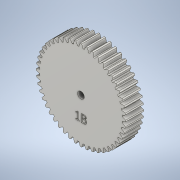
# Autodesk Inventor part: Spur Gear1
Saved by Autodesk Inventor 2021 (Build 250183000, 183)
## iProperties
CustomPartVersion: 0
Created: 2021-04-14
Part Number: Spur Gear1
Material: Steel
Document SubType Name: Modeling
Designer: Nabeel Azafer
Categories: <?xml version="1.0" encoding="UTF-16"?> <MemberInstance><Categories><FamilyTemplate><FamilyTemplateParameter ValueType="xs:double" Id="1" ObjectReferenceKey="da_z" ObjectType="kUserParameterObject"/><FamilyTemplateParameter ValueType="xs:double" Id="2" ObjectReferenceKey="da_b" ObjectType="kUserParameterObject"/><FamilyTemplateParameter ValueType="xs:double" Id="3" ObjectReferenceKey="da_beta" ObjectType="kUserParameterObject"/><FamilyTemplateParameter ValueType="xs:double" Id="4" ObjectReferenceKey="da_da" ObjectType="kUserParameterObject"/><FamilyTemplateParameter ValueType="xs:double" Id="5" ObjectReferenceKey="da_aw" ObjectType="kUserParameterObject"/><FamilyTemplateParameter ValueType="xs:string" Id="6" ObjectReferenceKey="EAIAABAAAACIAQAAAAAAAIAAAAAAAAAA" ObjectType="83910656" SubObjectId="SurfaceGeometry"/></FamilyTemplate><ParamToTemplateMap><ParamToTemplate CategoryParameter="//CategoryParameter[@InternalName='046C89C9-8512-4d59-83FE-43B91F4F132A']" TemplateParameter="1"/><ParamToTemplate CategoryParameter="//CategoryParameter[@InternalName='2552DF32-E462-4b46-AEBF-C6C7768E72AC']" TemplateParameter="2"/><ParamToTemplate CategoryParameter="//CategoryParameter[@InternalName='C9EE641D-15FC-4fae-A226-E94C4372FDD7']" TemplateParameter="3"/><ParamToTemplate><ParamToTemplate CategoryParameter="//CategoryParameter[@InternalName='00B6519A-459B-49c7-AD84-2E56D39A5744']" ConstantValue="0.000000"/></ParamToTemplate><ParamToTemplate><ParamToTemplate CategoryParameter="//CategoryParameter[@InternalName='04B31F0E-C7A6-4894-AA32-9629BEFACF47']" ConstantValue="0.800000"/></ParamToTemplate><ParamToTemplate><ParamToTemplate CategoryParameter="//CategoryParameter[@InternalName='43CBEC2E-7847-49e7-A936-2F7889FCB2D9']" ConstantValue="0.350000"/></ParamToTemplate><ParamToTemplate><ParamToTemplate CategoryParameter="//CategoryParameter[@InternalName='B1EFC894-105D-4ebd-86BF-FA20ED196853']" ConstantValue="0.500000"/></ParamToTemplate><ParamToTemplate><ParamToTemplate CategoryParameter="//CategoryParameter[@InternalName='51175063-3D10-4879-93E8-6246FE8B403D']" ConstantValue="2060000000.000000"/></ParamToTemplate><ParamToTemplate><ParamToTemplate CategoryParameter="//CategoryParameter[@InternalName='A3A52E27-4454-46a9-B0BD-C932399B70AF']" ConstantValue="0.300000"/></ParamToTemplate><ParamToTemplate><ParamToTemplate CategoryParameter="//CategoryParameter[@InternalName='91B76062-C214-41d9-B1B9-14D2AB99603D']" ConstantValue="0.080000"/></ParamToTemplate><ParamToTemplate><ParamToTemplate CategoryParameter="//CategoryParameter[@InternalName='374E806E-8B8A-4dda-A9AA-1039D6500AD2']" ConstantValue="12.500000"/></ParamToTemplate><ParamToTemplate><ParamToTemplate CategoryParameter="//CategoryParameter[@InternalName='2D373A89-B862-43d6-8D0B-0CBF12AB9F6C']" ConstantValue="0.349066"/></ParamToTemplate><ParamToTemplate CategoryParameter="//CategoryParameter[@InternalName='37777632-D6A2-4fac-9D53-DB8ACD95C989']" TemplateParameter="4"/><ParamToTemplate CategoryParameter="//CategoryParameter[@InternalName='FD1017F1-B727-4f7e-9707-0F86F1FF9423']" TemplateParameter="5"/><ParamToTemplate><ParamToTemplate CategoryParameter="//CategoryParameter[@InternalName='9E1B4470-B2D3-4ff1-B813-535BB4CDF51A']" ConstantValue="3520000.000000"/></ParamToTemplate><ParamToTemplate><ParamToTemplate CategoryParameter="//CategoryParameter[@InternalName='F8452263-BFF6-458c-9FB1-07C4B99E95CD']" ConstantValue="11400000.000000"/></ParamToTemplate><ParamToTemplate><ParamToTemplate CategoryParameter="//CategoryParameter[@InternalName='3E3BB259-FD49-497f-8171-6EBC954A3479']" ConstantValue="2.000000"/></ParamToTemplate><ParamToTemplate CategoryParameter="//CategoryParameter[@InternalName='27C3BAF2-7550-4e4b-AE2C-0DB134B7D9B7']" TemplateParameter="6"/></ParamToTemplateMap><Category DisplayName="Gear" InternalName="DC85795E-93AB-48d5-8EEE-5A27447B64BD" Mnemonic="Gear"><CategoryParameter DisplayName="z" InternalName="046C89C9-8512-4d59-83FE-43B91F4F132A" Mnemonic="z"/><CategoryParameter DisplayName="b" InternalName="2552DF32-E462-4b46-AEBF-C6C7768E72AC" Mnemonic="b"/><CategoryParameter DisplayName="||b|" InternalName="C9EE641D-15FC-4fae-A226-E94C4372FDD7" Mnemonic="beta"/><CategoryParameter DisplayName="x" InternalName="00B6519A-459B-49c7-AD84-2E56D39A5744" Mnemonic="x"/><CategoryParameter DisplayName="a*" InternalName="04B31F0E-C7A6-4894-AA32-9629BEFACF47" Mnemonic="a"/><CategoryParameter DisplayName="c*" InternalName="43CBEC2E-7847-49e7-A936-2F7889FCB2D9" Mnemonic="c"/><CategoryParameter DisplayName="r|.f|*" InternalName="B1EFC894-105D-4ebd-86BF-FA20ED196853" Mnemonic="rf"/><CategoryParameter DisplayName="E" InternalName="51175063-3D10-4879-93E8-6246FE8B403D" Mnemonic="E"/><CategoryParameter DisplayName="||m|" InternalName="A3A52E27-4454-46a9-B0BD-C932399B70AF" Mnemonic="mi"/><Category DisplayName="SpurGear" InternalName="26C5A22E-A91E-4dfd-A3B3-23CCAFAE1764" Mnemonic="SpurGear"><CategoryParameter DisplayName="m" InternalName="91B76062-C214-41d9-B1B9-14D2AB99603D" Mnemonic="m"/><CategoryParameter DisplayName="P" InternalName="374E806E-8B8A-4dda-A9AA-1039D6500AD2" Mnemonic="PP"/><CategoryParameter DisplayName="||a|" InternalName="2D373A89-B862-43d6-8D0B-0CBF12AB9F6C" Mnemonic="alpha"/><CategoryParameter DisplayName="d|.a|" InternalName="37777632-D6A2-4fac-9D53-DB8ACD95C989" Mnemonic="da"/><CategoryParameter DisplayName="a|.w|" InternalName="FD1017F1-B727-4f7e-9707-0F86F1FF9423" Mnemonic="aw"/><CategoryParameter DisplayName="||s||.Flim|" InternalName="9E1B4470-B2D3-4ff1-B813-535BB4CDF51A" Mnemonic="sFlim"/><CategoryParameter DisplayName="||s||.Hlim|" InternalName="F8452263-BFF6-458c-9FB1-07C4B99E95CD" Mnemonic="sHlim"/><CategoryParameter DisplayName="type" InternalName="3E3BB259-FD49-497f-8171-6EBC954A3479" Mnemonic="type"/><CategoryParameter DisplayName="PitchDiameter" InternalName="27C3BAF2-7550-4e4b-AE2C-0DB134B7D9B7" Mnemonic="IDS_PITCHDIAM"/></Category></Category></Categories></MemberInstance>
Density: 1 g/cm^3
Appearance: Steel
Author: Nabeel Azafer
Autodesk Inventor part; units mm, degrees
note: some values were not read from the file. Chosen so that the rebuilt part matches the saved one: direction of "Emboss1".
sketch "Sketch1" plane through (0, 0, 0) normal (0, 0, 1) x (1, 0, 0)
  circle A0 centre (0, 0) radius 19.84
  dimension "d0" = 39.68
  constraints: 1 centre point
  measures "d0" diameter of A0
extrude "Extrusion1" add sketch "Sketch1" along normal blind 8
ref_plane "Work Plane2" through (0, 0, 4) normal (0, 0, 1) x (1, 0, 0)
sketch "Sketch2" plane through (0, 0, 0) normal (0, 0, -1) x (-1, 0, 0)
  circle A0 centre (0, 0) radius 19.84 projected
  circle A1 centre (0, 0) radius 19.2
  dimension "d3" = 38.4
  constraints: 1 centre point, 1 coincident
  measures "d3" diameter of A1
surface extrude "Pitch Diameter" sketch "Sketch2" against normal through all shown no curves A1
ref_plane "Work Plane8" through (0, 0, 0) normal (0.9978589, 0.0654031, 0) x (0, 0, 1)
ref_plane "Work Plane9" through (0, 0, 0) normal (1, 0, 0) x (0, 1, 0)
spur gear teeth "Spur Gear" teeth 48 pitch diameter 38.4 tip diameter 39.68 root diameter 36.56 face width 8 start plane through (0, 0, 0) normal (0, 0, -1) x (-1, 0, 0)
sketch "Sketch3" plane through (0, 0, 8) normal (0, 0, 1) x (1, 0, 0)
  circle A0 centre (0, 0) radius 1.5
  dimension "d49" = 3
  constraints: 1 centre point, 1 coincident
  measures "d49" diameter of A0
hole "Hole1" at (0, 0, 8) direction (0, 0, -1) diameter 3 end through all
sketch "Sketch4" plane through (0, 0, 8) normal (0, 0, 1) x (1, 0, 0)
  line L0 (-2.832, -6.8426) -> (22.1505, -6.8426) construction
  line L1 (22.1505, -6.8426) -> (22.1505, -16.435) construction
  line L2 (22.1505, -16.435) -> (-2.832, -16.435) construction
  line L3 (-2.832, -16.435) -> (-2.832, -6.8426) construction
  line L4 (-0.5941, -10.3539) -> (-2.3016, -10.3539)
  line L5 (-2.3016, -10.3539) -> (-2.3016, -9.9966)
  line L6 (-2.3016, -9.9966) -> (-1.6663, -9.9966)
  line L7 (-1.6663, -9.9966) -> (-1.6663, -7.6509)
  line L8 (-1.6663, -7.6509) -> (-2.3016, -7.6509)
  line L9 (-2.3016, -7.6509) -> (-2.3016, -7.3304)
  spline S0 degree 2 poles (-2.3016, -7.3304) (-1.9414, -7.3304) (-1.601, -7.1262) (-1.5783, -6.8426) knots 0 0 0 1 2 2 2
  line L10 (-1.5783, -6.8426) -> (-1.2153, -6.8426)
  line L11 (-1.2153, -6.8426) -> (-1.2153, -9.9966)
  line L12 (-1.2153, -9.9966) -> (-0.5941, -9.9966)
  line L13 (-0.5941, -9.9966) -> (-0.5941, -10.3539)
  spline S1 degree 2 poles (2.523, -9.279) (2.523, -9.5399) (2.3244, -9.9398) (2.1599, -10.0703) knots 0 0 0 1 2 2 2
  spline S2 degree 2 poles (2.1599, -10.0703) (1.9614, -10.2235) (1.5104, -10.3539) (1.153, -10.3539) knots 0 0 0 1 2 2 2
  line L14 (1.153, -10.3539) -> (0.149, -10.3539)
  line L15 (0.149, -10.3539) -> (0.149, -6.8539)
  line L16 (0.149, -6.8539) -> (1.0764, -6.8539)
  spline S3 degree 2 poles (1.0764, -6.8539) (1.4508, -6.8539) (1.8252, -6.9022) (1.9954, -6.9958) knots 0 0 0 1 2 2 2
  spline S4 degree 2 poles (1.9954, -6.9958) (2.1854, -7.095) (2.3584, -7.4212) (2.3584, -7.6424) knots 0 0 0 1 2 2 2
  spline S5 degree 2 poles (2.3584, -7.6424) (2.3584, -7.8892) (2.0975, -8.2806) (1.8678, -8.3912) knots 0 0 0 1 2 2 2
  line L17 (1.8678, -8.3912) -> (1.8678, -8.4082)
  spline S6 degree 2 poles (1.8678, -8.4082) (2.1798, -8.4933) (2.523, -8.9443) (2.523, -9.279) knots 0 0 0 1 2 2 2
  spline S7 degree 2 poles (2.0379, -9.2988) (2.0379, -9.1003) (1.9245, -8.845) (1.7543, -8.7543) knots 0 0 0 1 2 2 2
  spline S8 degree 2 poles (1.7543, -8.7543) (1.6437, -8.6975) (1.3828, -8.6635) (1.1417, -8.6635) knots 0 0 0 1 2 2 2
  line L18 (1.1417, -8.6635) -> (0.6141, -8.6635)
  line L19 (0.6141, -8.6635) -> (0.6141, -9.9569)
  line L20 (0.6141, -9.9569) -> (0.9913, -9.9569)
  spline S9 degree 2 poles (0.9913, -9.9569) (1.2977, -9.9569) (1.6494, -9.9001) (1.7855, -9.8094) knots 0 0 0 1 2 2 2
  spline S10 degree 2 poles (1.7855, -9.8094) (1.916, -9.7158) (2.0379, -9.4832) (2.0379, -9.2988) knots 0 0 0 1 2 2 2
  spline S11 degree 2 poles (1.8734, -7.7077) (1.8734, -7.5829) (1.7884, -7.3957) (1.6948, -7.3418) knots 0 0 0 1 2 2 2
  spline S12 degree 2 poles (1.6948, -7.3418) (1.5813, -7.2794) (1.3062, -7.251) (1.0594, -7.251) knots 0 0 0 1 2 2 2
  line L21 (1.0594, -7.251) -> (0.6141, -7.251)
  line L22 (0.6141, -7.251) -> (0.6141, -8.2749)
  line L23 (0.6141, -8.2749) -> (1.1417, -8.2749)
  spline S13 degree 2 poles (1.1417, -8.2749) (1.3601, -8.2749) (1.5671, -8.2295) (1.6777, -8.1586) knots 0 0 0 1 2 2 2
  spline S14 degree 2 poles (1.6777, -8.1586) (1.7855, -8.0906) (1.8734, -7.8722) (1.8734, -7.7077) knots 0 0 0 1 2 2 2
  point P0 (0, 0)
  constraints: 2 other
emboss "Emboss1" sketch "Sketch4" operation cut depth 1 direction (0, 0, -1)
equation "\"d0\" = da_da"
equation "\"d1\" = da_b"
equation "\"d3\" = da_d"
equation "\"d16\" = da_aw"
equation "\"d43\" = da_aw"
equation "\"d46\" = da_aw"
equation "\"da_da\" = 39.68"
equation "\"da_b\" = 8"
equation "\"da_d\" = 38.4"
equation "\"da_aw\" = 28.8"
body "Solid1"
body "Srf1"
